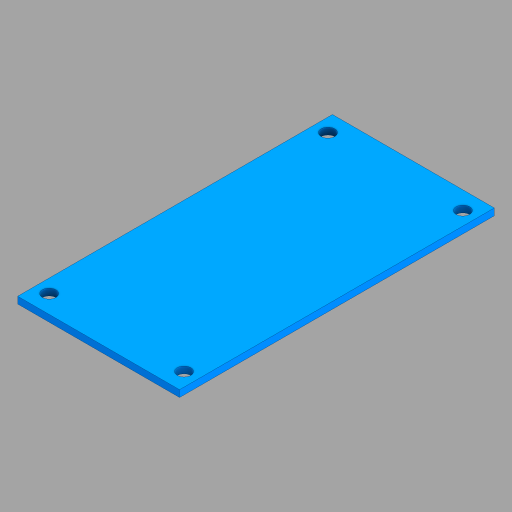
# Autodesk Inventor part: DC-DC
Saved by Autodesk Inventor 2024.2 (Build 282272000, 272)
## iProperties
Created: 2024-01-20
Part Number: DC-DC
Material: Типовые
Document SubType Name: Modeling
Designer: Fedor Orlov
Density: 1 g/cm^3
Appearance: По умолчанию
Author: Fedor Orlov
Autodesk Inventor part; units mm, degrees
ref_plane "YZ Plane" through (0, 0, 0) normal (1, 0, 0) x (0, 1, 0)
ref_plane "XZ Plane" through (0, 0, 0) normal (0, 1, 0) x (-1, 0, 0)
ref_plane "XY Plane" through (0, 0, 0) normal (0, 0, 1) x (1, 0, 0)
sketch "Эскиз1" plane through (0, 0, 0) normal (0, 1, 0) x (-1, 0, 0)
  line L0 (-18, -35) -> (18, -35)
  line L1 (18, -35) -> (18, 35)
  line L2 (18, 35) -> (-18, 35)
  line L3 (-18, 35) -> (-18, -35)
  line L4 (-18, -35) -> (18, 35) construction
  line L5 (18, -35) -> (-18, 35) construction
  line L6 (-15, -31) -> (15, -31) construction
  line L7 (15, -31) -> (15, 31) construction
  line L8 (15, 31) -> (-15, 31) construction
  line L9 (-15, 31) -> (-15, -31) construction
  line L10 (-15, -31) -> (15, 31) construction
  line L11 (15, -31) -> (-15, 31) construction
  circle A0 centre (15, 31) radius 1.5
  circle A1 centre (15, -31) radius 1.5
  circle A2 centre (-15, -31) radius 1.5
  circle A3 centre (-15, 31) radius 1.5
  point P0 (0, 0)
  dimension "d0" = 36
  dimension "d1" = 70
  dimension "d2" = 62
  dimension "d3" = 30
  dimension "d4" = 3
  dimension "d5" = 3
  dimension "d6" = 3
  dimension "d7" = 3
  constraints: 24 end point, 4 centre point, 4 coincident, 4 midpoint, 4 parallel, 2 horizontal, 2 perpendicular
  measures "d0" distance of L2.end L1.end
  measures "d1" distance of L1.end L0.end
  measures "d2" distance of L6.end L7.end
  measures "d3" distance of L6.start L6.end
  measures "d4" diameter of A0
  measures "d5" diameter of A1
  measures "d6" diameter of A2
  measures "d7" diameter of A3
extrude "Выдавливание1" add sketch "Эскиз1" along normal blind 1.5
